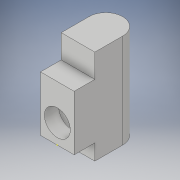
# Autodesk Inventor part: Wrist1-lrg
Saved by Autodesk Inventor 2017 (Build 210142000, 142)
## iProperties
Created: 2017-05-25
Part Number: Wrist1-lrg
Material: Generic
Document SubType Name: Modeling
Designer: garre
Density: 1 g/cm^3
Appearance: Default
Author: garre
Autodesk Inventor part; units mm, degrees
ref_plane "YZ Plane" through (0, 0, 0) normal (1, 0, 0) x (0, 1, 0)
ref_plane "XZ Plane" through (0, 0, 0) normal (0, 1, 0) x (-1, 0, 0)
ref_plane "XY Plane" through (0, 0, 0) normal (0, 0, 1) x (1, 0, 0)
sketch "Sketch1" plane through (0, 0, 0) normal (0, 0, 1) x (1, 0, 0)
  circle A0 centre (0, 0) radius 25.4
  line L0 (-33.02, -38.1) -> (33.02, -38.1)
  line L1 (33.02, -38.1) -> (33.02, 69.85)
  line L2 (33.02, 69.85) -> (-33.02, 69.85)
  line L3 (-33.02, 69.85) -> (-33.02, -38.1)
  dimension "d0" = 50.8
  dimension "d1" = 66.04
  dimension "d2" = 107.95
  dimension "d3" = 33.02
  dimension "d4" = 38.1
  constraints: 8 end point, 2 parallel, 1 centre point, 1 coincident, 1 horizontal, 1 perpendicular
  measures "d0" diameter of A0
  measures "d1" distance of L0.start L0.end
  measures "d2" distance of L0.end L1.end
  measures "d3" distance from line of L1 point (0, 0)
  measures "d4" distance from line of L0 point (0, 0)
extrude "Extrusion1" add sketch "Sketch1" against normal blind 40.64
sketch "Sketch2" plane through (0, 0, -40.64) normal (0, 0, -1) x (-1, 0, 0)
  circle A0 centre (0, 0) radius 25.1006
  constraints: 1 centre point, 1 coincident
extrude "Extrusion2" add sketch "Sketch2" against normal blind 12.7
sketch "Sketch3" plane through (-33.02, -38.1, 0) normal (0, -1, 0) x (1, 0, 0)
  line L0 (0, 0) -> (66.04, 0) projected
  line L1 (66.04, 0) -> (0, 0)
  line L2 (0, 0) -> (0, -95.25)
  line L3 (0, -95.25) -> (66.04, -95.25)
  line L4 (66.04, -95.25) -> (66.04, 0)
  line L5 (66.04, -40.64) -> (0, -40.64)
  arc A0 (0, -95.25) -> (66.04, -95.25) centre (33.02, -95.25) ccw
  line L6 (0, -40.64) -> (66.04, -40.64) projected
  line L7 (0, -40.64) -> (66.04, -40.64)
  line L8 (66.04, -40.64) -> (66.04, -95.25)
  line L9 (66.04, -95.25) -> (0, -95.25)
  line L10 (0, -95.25) -> (0, -40.64)
  point P0 (33.02, 0)
  dimension "d9" = 54.61
  constraints: 18 end point, 4 parallel, 3 perpendicular, 2 horizontal, 2 point on circle, 2 tangent, 1 centre point, 1 point on line
  measures "d9" distance between parallel lines of L3 L5
extrude "Extrusion3" add sketch "Sketch3" along normal mid plane 62.23 contours L5 L4 L3 L2 | L3 A0
sketch "Sketch4" plane through (-33.02, -38.1, 0) normal (0, -1, 0) x (1, 0, 0)
  point P0 (33.02, 0)
sketch "Sketch5" plane through (-33.02, -6.985, 0) normal (0, 1, 0) x (1, 0, 0)
  arc A0 (66.04, 95.25) -> (0, 95.25) centre (33.02, 95.25) ccw projected
  line L0 (66.04, 40.64) -> (66.04, 95.25) projected
  line L1 (0, 95.25) -> (66.04, 95.25)
  line L2 (66.04, 95.25) -> (66.04, 40.64)
  line L3 (66.04, 40.64) -> (0, 40.64)
  line L4 (0, 40.64) -> (0, 95.25)
  arc A1 (66.04, 95.25) -> (0, 95.25) centre (33.02, 95.25) ccw
  point P0 (33.02, 0)
  constraints: 8 end point, 2 parallel, 2 point on circle, 2 tangent, 1 centre point, 1 horizontal, 1 perpendicular
extrude "Extrusion4" add sketch "Sketch5" along normal blind 123.19
sketch "Sketch6" plane through (-33.02, -69.215, 0) normal (0, -1, 0) x (1, 0, 0)
  arc A0 (0, -95.25) -> (66.04, -95.25) centre (33.02, -95.25) ccw projected
  line L0 (0, -95.25) -> (33.02, -95.25)
  circle A1 centre (33.02, -95.25) radius 26.67
  point P0 (33.02, 0)
  dimension "d16" = 53.34
  constraints: 2 end point, 1 centre point, 1 coincident, 1 horizontal
  measures "d16" diameter of A1
extrude "Extrusion5" cut sketch "Sketch6" against normal blind 60.96
equation "\"d3\" = 0.5 * d1"
body "Solid1"
